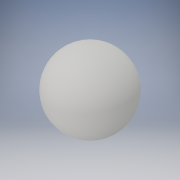
# Autodesk Inventor part: Power Cell
Saved by Autodesk Inventor 2019.4 (Build 234330000, 330)
## iProperties
Created: 2020-01-06
Part Number: Power Cell
Material: Generic
Document SubType Name: Modeling
Designer: admin
Appearance: Default
Surface Area: 993.147 cm^2
Volume: 2943.02 cm^3
Author: admin
Autodesk Inventor part; units mm, degrees
ref_plane "YZ Plane" through (0, 0, 0) normal (1, 0, 0) x (0, 1, 0)
ref_plane "XZ Plane" through (0, 0, 0) normal (0, 1, 0) x (-1, 0, 0)
ref_plane "XY Plane" through (0, 0, 0) normal (0, 0, 1) x (1, 0, 0)
sketch "Sketch1" plane through (0, 0, 0) normal (1, 0, 0) x (0, 1, 0)
  arc A0 (88.9, 0) -> (-88.9, 0) centre (0, 0) ccw
  line L0 (88.9, 0) -> (-88.9, 0)
  arc A1 (-88.9, 0) -> (88.9, 0) centre (0, 0) ccw construction
  dimension "d0" = 177.8
  constraints: 4 point on circle, 2 centre point, 2 end point, 1 coincident, 1 horizontal, 1 line through centre
  measures "d0" diameter of A0
revolve "Revolution1" add sketch "Sketch1" angle 360 about axis through (0, 88.9, 0) along (0, -1, 0)
body "Solid1"
